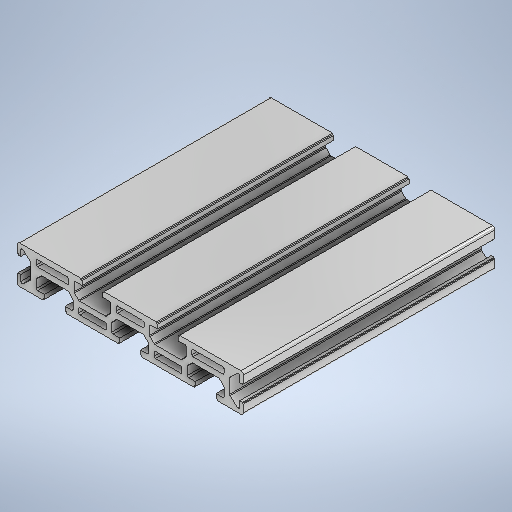
# Autodesk Inventor part: Perfil 15×90 7 rasgos_001
Saved by Autodesk Inventor 2026 (Build 300175000, 175)
## iProperties
Created: 2025-04-03
Part Number: Perfil 15×90 7 rasgos_001
Material: Aluminum 6061
Document SubType Name: Modeling
Designer: Carlos Dias
Density: 2.7 g/cm^3
Appearance: Aluminum - Polished
Author: Carlos Dias
Autodesk Inventor part; units mm, degrees
sketch "Sketch2" plane through (0, 0, 0) normal (0, 0, 1) x (1, 0, 0)
  line L0 (-15, 15) -> (0, 15) construction
  line L1 (-30, 15) -> (0, 15) construction
  line L2 (-45, 15) -> (0, 15) construction
  line L3 (-45, 15) -> (-45, 0) construction
  arc A0 (-44, 15) -> (-45, 14) centre (-44, 14) ccw
  line L4 (-45, 10.6) -> (-45, 4.4) construction
  arc A1 (-45, 1) -> (-44, 0) centre (-44, 1) ccw
  line L5 (-45, 0) -> (0, 0) construction
  line L6 (-45, 4.4) -> (-43.5, 4.4) construction
  line L7 (-45, 10.6) -> (-43.5, 10.6) construction
  line L8 (-45, 10.6) -> (-44.6, 10.6) construction
  line L9 (-44.6, 10.6) -> (-44.6, 11)
  line L10 (-44.6, 11) -> (-45, 11)
  line L11 (-45, 11) -> (-45, 10.6) construction
  line L12 (-45, 14) -> (-45, 11)
  line L13 (-44.6, 10.6) -> (-43.5, 10.6)
  line L14 (-43.5, 14.1024) -> (-43.5, 10.6) construction
  line L15 (-39.5, 10.6) -> (-39.5, 4.4) construction
  line L16 (-45, 4.4) -> (-44.6, 4.4) construction
  line L17 (-44.6, 4.4) -> (-44.6, 4)
  line L18 (-44.6, 4) -> (-45, 4)
  line L19 (-45, 4) -> (-45, 4.4) construction
  line L20 (-45, 4) -> (-45, 1)
  line L21 (-44.6, 4.4) -> (-43.5, 4.4)
  line L22 (-43.5, 4.4) -> (-43.5, 0.8976) construction
  line L23 (-43.5, 0.8976) -> (-39.5, 4.4) construction
  line L24 (-43.5, 14.1024) -> (-39.5, 10.6) construction
  line L25 (-34.1, 0) -> (-34.6, 0) construction
  line L26 (-34.6, 0) -> (-34.6, 0.5)
  line L27 (-34.6, 0.5) -> (-34.1, 0.5)
  line L28 (-34.1, 0.5) -> (-34.1, 0) construction
  line L29 (-44, 0) -> (-34.6, 0)
  arc A2 (-42.6706, 13.3762) -> (-43.5, 13) centre (-43, 13) ccw
  arc A3 (-43.5, 2) -> (-42.6706, 1.6238) centre (-43, 2) ccw
  line L30 (-43.5, 13) -> (-43.5, 10.6)
  line L31 (-43, 13.5) -> (-43.5, 13.5) construction
  line L32 (-43.5, 4.4) -> (-43.5, 2)
  arc A4 (-39.5, 10.3732) -> (-39.6706, 10.7494) centre (-40, 10.3732) ccw
  arc A5 (-39.6706, 4.2506) -> (-39.5, 4.6268) centre (-40, 4.6268) ccw
  line L33 (-39.5, 10.3732) -> (-39.5, 4.6268)
  line L34 (-42.6706, 13.3762) -> (-39.6706, 10.7494)
  line L35 (-39.6706, 4.2506) -> (-42.6706, 1.6238)
  line L36 (-34.1, 2.2) -> (-34.1, 0.5)
  line L37 (-37.3, 2.2) -> (-34.1, 2.2) construction
  line L38 (-37.3, 6.1444) -> (-37.3, 2.2) construction
  line L39 (-44, 15) -> (-19.1, 15) construction
  line L40 (-37.3, 12.8) -> (-24.5, 12.8) construction
  line L41 (-37.3, 10.3) -> (-24.5, 10.3) construction
  line L42 (-19.1, 15) -> (-19.1, 12.8) construction
  line L43 (-19.1, 15) -> (-19.6, 15) construction
  line L44 (-19.6, 15) -> (-19.6, 14.5)
  line L45 (-19.6, 14.5) -> (-19.1, 14.5)
  line L46 (-19.1, 14.5) -> (-19.1, 15) construction
  line L47 (-19.1, 14.5) -> (-19.1, 12.8)
  line L48 (-35.3444, 8.1) -> (-37.3, 6.1444) construction
  line L49 (-35.3444, 8.1) -> (-30, 8.1) construction
  line L50 (-30, 8.1) -> (-24.6556, 8.1) construction
  line L51 (-24.6556, 8.1) -> (-22.7, 6.1444) construction
  line L52 (-22.7, 6.1444) -> (-22.7, 2.2) construction
  line L53 (-22.7, 2.2) -> (-25.9, 2.2) construction
  line L54 (-25.9, 2.2) -> (-25.9, 0) construction
  line L55 (-25.9, 0) -> (-25.4, 0) construction
  line L56 (-25.4, 0) -> (-25.4, 0.5)
  line L57 (-25.4, 0.5) -> (-25.9, 0.5)
  line L58 (-25.9, 0.5) -> (-25.9, 0) construction
  line L59 (-25.9, 2.2) -> (-25.9, 0.5)
  line L60 (-22.3, 12.8) -> (-19.1, 12.8) construction
  line L61 (-22.3, 12.8) -> (-22.3, 8.8556) construction
  line L62 (-22.3, 8.8556) -> (-20.3444, 6.9) construction
  line L63 (-20.3444, 6.9) -> (-15, 6.9) construction
  line L64 (-15, 6.9) -> (-9.6556, 6.9) construction
  line L65 (-7.7, 8.8556) -> (-9.6556, 6.9) construction
  line L66 (-7.7, 12.8) -> (-7.7, 8.8556) construction
  line L67 (-10.9, 12.8) -> (-7.7, 12.8) construction
  line L68 (-37.3, 12.8) -> (-37.3, 10.3) construction
  arc A6 (-36.8, 12.8) -> (-37.3, 12.3) centre (-36.8, 12.3) ccw
  arc A7 (-37.3, 10.8) -> (-36.8, 10.3) centre (-36.8, 10.8) ccw
  line L69 (-37.3, 12.3) -> (-37.3, 10.8)
  line L70 (-24.5, 12.8) -> (-24.5, 10.3) construction
  arc A8 (-25, 10.3) -> (-24.5, 10.8) centre (-25, 10.8) ccw
  arc A9 (-24.5, 12.3) -> (-25, 12.8) centre (-25, 12.3) ccw
  line L71 (-24.5, 12.3) -> (-24.5, 10.8)
  line L72 (-25, 12.8) -> (-36.8, 12.8)
  line L73 (-25, 10.3) -> (-36.8, 10.3)
  line L74 (-10.9, 15) -> (-10.9, 12.8) construction
  line L75 (-10.9, 15) -> (-10.4, 15) construction
  line L76 (-10.4, 15) -> (-10.4, 14.5)
  line L77 (-10.4, 14.5) -> (-10.9, 14.5)
  line L78 (-10.9, 14.5) -> (-10.9, 15) construction
  line L79 (-10.9, 14.5) -> (-10.9, 12.8)
  line L80 (-19.6, 15) -> (-44, 15)
  line L81 (-20.5, 4.7) -> (-9.5, 4.7) construction
  line L82 (-9.5, 4.7) -> (-9.5, 2.2) construction
  line L83 (-9.5, 2.2) -> (-20.5, 2.2) construction
  line L84 (-20.5, 2.2) -> (-20.5, 4.7) construction
  line L85 (-4.1, 0) -> (-4.1, 2.2) construction
  line L86 (-7.3, 2.2) -> (-4.1, 2.2) construction
  line L87 (-7.3, 6.1444) -> (-7.3, 2.2) construction
  arc A10 (-20, 4.7) -> (-20.5, 4.2) centre (-20, 4.2) ccw
  arc A11 (-20.5, 2.7) -> (-20, 2.2) centre (-20, 2.7) ccw
  arc A12 (-9.5, 4.2) -> (-10, 4.7) centre (-10, 4.2) ccw
  arc A13 (-10, 2.2) -> (-9.5, 2.7) centre (-10, 2.7) ccw
  line L88 (-9.5, 4.2) -> (-9.5, 2.7)
  line L89 (-20, 2.2) -> (-10, 2.2)
  line L90 (-20, 4.7) -> (-10, 4.7)
  line L91 (-20.5, 4.2) -> (-20.5, 2.7)
  line L92 (-5.3444, 8.1) -> (-7.3, 6.1444) construction
  line L93 (-5.3444, 8.1) -> (0, 8.1) construction
  line L94 (-4.1, 0) -> (-4.6, 0) construction
  line L95 (-4.6, 0) -> (-4.6, 0.5)
  line L96 (-4.6, 0.5) -> (-4.1, 0.5)
  line L97 (-4.1, 0.5) -> (-4.1, 0) construction
  line L98 (-4.6, 0) -> (-25.4, 0)
  line L99 (-4.1, 2.2) -> (-4.1, 0.5)
  line L100 (-10.4, 15) -> (0, 15)
  line L101 (-5.5, 12.8) -> (0, 12.8) construction
  line L102 (-5.5, 10.3) -> (0, 10.3) construction
  line L103 (-5.5, 12.8) -> (-5.5, 10.3) construction
  arc A14 (-5, 12.8) -> (-5.5, 12.3) centre (-5, 12.3) ccw
  arc A15 (-5.5, 10.8) -> (-5, 10.3) centre (-5, 10.8) ccw
  line L104 (-5.5, 12.3) -> (-5.5, 10.8)
  line L105 (-5, 12.8) -> (0, 12.8)
  line L106 (-5, 10.3) -> (0, 10.3)
  line L107 (0, 15) -> (0, 0)
  arc A16 (-37.3, 2.7) -> (-36.8, 2.2) centre (-36.8, 2.7) ccw
  arc A17 (-37.1536, 6.2908) -> (-37.3, 5.9373) centre (-36.8, 5.9373) ccw
  line L108 (-37.3, 5.9373) -> (-37.3, 2.7)
  line L109 (-36.8, 2.2) -> (-34.1, 2.2)
  arc A18 (-35.1373, 8.1) -> (-35.4908, 7.9536) centre (-35.1373, 7.6) ccw
  line L110 (-35.4908, 7.9536) -> (-37.1536, 6.2908)
  arc A19 (-24.5092, 7.9536) -> (-24.8627, 8.1) centre (-24.8627, 7.6) ccw
  line L111 (-35.1373, 8.1) -> (-24.8627, 8.1)
  arc A20 (-22.7, 5.9373) -> (-22.8464, 6.2908) centre (-23.2, 5.9373) ccw
  line L112 (-24.5092, 7.9536) -> (-22.8464, 6.2908)
  arc A21 (-23.2, 2.2) -> (-22.7, 2.7) centre (-23.2, 2.7) ccw
  line L113 (-22.7, 5.9373) -> (-22.7, 2.7)
  line L114 (-25.9, 2.2) -> (-23.2, 2.2)
  arc A22 (-21.8, 12.8) -> (-22.3, 12.3) centre (-21.8, 12.3) ccw
  arc A23 (-22.3, 9.0627) -> (-22.1536, 8.7092) centre (-21.8, 9.0627) ccw
  arc A24 (-20.4908, 7.0464) -> (-20.1373, 6.9) centre (-20.1373, 7.4) ccw
  arc A25 (-9.8627, 6.9) -> (-9.5092, 7.0464) centre (-9.8627, 7.4) ccw
  arc A26 (-7.8464, 8.7092) -> (-7.7, 9.0627) centre (-8.2, 9.0627) ccw
  arc A27 (-7.7, 12.3) -> (-8.2, 12.8) centre (-8.2, 12.3) ccw
  line L115 (-19.1, 12.8) -> (-21.8, 12.8)
  line L116 (-22.3, 12.3) -> (-22.3, 9.0627)
  line L117 (-22.1536, 8.7092) -> (-20.4908, 7.0464)
  line L118 (-20.1373, 6.9) -> (-9.8627, 6.9)
  line L119 (-7.8464, 8.7092) -> (-9.5092, 7.0464)
  line L120 (-7.7, 12.3) -> (-7.7, 9.0627)
  line L121 (-10.9, 12.8) -> (-8.2, 12.8)
  arc A28 (-7.3, 2.7) -> (-6.8, 2.2) centre (-6.8, 2.7) ccw
  arc A29 (-7.1536, 6.2908) -> (-7.3, 5.9373) centre (-6.8, 5.9373) ccw
  arc A30 (-5.1373, 8.1) -> (-5.4908, 7.9536) centre (-5.1373, 7.6) ccw
  line L122 (-4.1, 2.2) -> (-6.8, 2.2)
  line L123 (-7.3, 5.9373) -> (-7.3, 2.7)
  line L124 (-5.4908, 7.9536) -> (-7.1536, 6.2908)
  line L125 (-5.1373, 8.1) -> (0, 8.1)
  point P0 (-45, 7.5)
  point P1 (-39.5, 7.5)
  point P2 (-30.9, 12.8)
  point P3 (-37.3, 11.55)
  point P4 (-20.7, 12.8)
  point P5 (-22.3, 10.8278)
  point P6 (-24.5, 11.55)
  point P7 (-21.3222, 7.8778)
  point P8 (-22.7, 4.1722)
  point P9 (-20.5, 3.45)
  point P10 (-9.5, 3.45)
  point P11 (-7.3, 4.1722)
  point P12 (-7.7, 10.8278)
  point P13 (-30.9, 12.8)
  point P14 (-2.75, 12.8)
  dimension "d2" = 15
  dimension "d3" = 15
  dimension "d4" = 30
  dimension "d5" = 45
  dimension "d6" = 1
  dimension "d7" = 6.2
  dimension "d8" = 1.5
  dimension "d9" = 0.4
  dimension "d11" = 5.5
  dimension "d12" = 6.2
  dimension "d13" = 4.1
  dimension "d15" = 0.5
  dimension "d16" = 0.5
  dimension "d18" = 1.5
  dimension "d19" = 2.2
  dimension "d20" = 2.2
  dimension "d23" = 2.5
  dimension "d26" = 4.1
  dimension "d29" = 135
  dimension "d30" = 2.2
  dimension "d31" = 135
  dimension "d33" = 4.1
  dimension "d38" = 135
  dimension "d40" = 2.2
  dimension "d41" = 2.2
  dimension "d42" = 2.2
  dimension "d45" = 4.1
  dimension "d46" = 2.2
  dimension "d47" = 2.2
  dimension "d48" = 135
  dimension "d50" = 2.2
  constraints: 252 end point, 64 point on line, 63 tangent, 62 point on circle, 41 horizontal, 33 equal length, 31 centre point, 30 vertical, 29 equal radius, 17 midpoint, 16 parallel, 10 perpendicular, 10 vertical alignment, 5 horizontal alignment, 1 coincident, 1 collinear
  measures "d2" distance of point (0, 0) L0.end
  measures "d3" distance of L0.start L0.end
  measures "d4" distance of L1.start L0.end
  measures "d5" distance of L2.start L0.end
  measures "d6" radius of A0
  measures "d7" distance of L4.start L4.end
  measures "d8" distance of L4.end L6.end
  measures "d9" distance of L9.end L10.end
  measures "d11" distance of L4.start L15.start
  measures "d12" distance of L15.start L15.end
  measures "d13" horizontal distance of L1.start L25.start
  measures "d15" distance of L25.end L26.end
  measures "d16" radius of A2
  measures "d18" distance between parallel lines of L2 L31
  measures "d19" distance of L36.start L25.start
  measures "d20" distance between parallel lines of L33 L38
  measures "d23" distance between parallel lines of L41 L40
  measures "d26" distance of L0.start L39.end
  measures "d29" angle of L49 L48
  measures "d30" distance between parallel lines of L41 L49
  measures "d31" angle of L50 L51
  measures "d33" horizontal distance of L1.start L53.end
  measures "d38" angle of L64 L65
  measures "d40" horizontal distance of point (-22.3, 10.828) point (-24.5, 11.55)
  measures "d41" distance from line of point (-21.322, 7.878) L51
  measures "d42" horizontal distance of point (-22.7, 4.172) point (-20.5, 3.45)
  measures "d45" distance of point (0, 0) L85.start
  measures "d46" horizontal distance of point (-9.5, 3.45) point (-7.3, 4.172)
  measures "d47" distance between parallel lines of L63 L81
  measures "d48" angle of L62 L63
  measures "d50" distance from line of point (-7.7, 10.828) L103
extrude "Extrusion1" add sketch "Sketch2" along normal mid plane 100 contours L80 L44 L45 L47 L115 A22 L116 A23 L117 A24 L118 A25 L119 A26 L120 A27 L121 L79 L77 L76 L100 L107 L105 A14 L104 A15 L106 L125 A30 L124 A29 L123 A28 L122 L99 L96 L95 L98 L56 L57 L59 L114 A21 L113 A20 L112 A19 L111 A18 L110 A17 L108 A16 L109 L36 L27 L26 L29 A1 L20 L18 L17 L21 L32 A3 L35 A5 L33 A4 L34 A2 L30 L13 L9 L10 L12 A0
mirror "Mirror1" about plane through (0, 0, 0) normal (1, 0, 0) of "Extrusion1"
equation "\"d20\" = d19"
body "Solid1"
